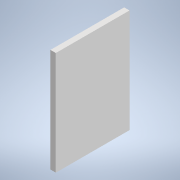
# Autodesk Inventor part: backPlate
Saved by Autodesk Inventor 2021.2 (Build 252289000, 289)
## iProperties
Created: 2021-02-12
Part Number: backPlate
Material: PC/ABS Plastic
Document SubType Name: Modeling
Designer: robst
Density: 0.357273 g/cm^3
Appearance: Smooth - White
Author: robst
Autodesk Inventor part; units mm, degrees
ref_plane "YZ Plane" through (0, 0, 0) normal (1, 0, 0) x (0, 1, 0)
ref_plane "XZ Plane" through (0, 0, 0) normal (0, 1, 0) x (-1, 0, 0)
ref_plane "XY Plane" through (0, 0, 0) normal (0, 0, 1) x (1, 0, 0)
sketch "Sketch1" plane through (0, 0, 0) normal (1, 0, 0) x (0, 1, 0)
  line L0 (-18.3138, 13.0328) -> (-18.3138, -13.0328)
  line L1 (-18.3138, -13.0328) -> (18.3138, -13.0328)
  line L2 (18.3138, -13.0328) -> (18.3138, 13.0328)
  line L3 (18.3138, 13.0328) -> (-18.3138, 13.0328)
  line L4 (-18.3138, 13.0328) -> (18.3138, -13.0328) construction
  line L5 (-18.3138, -13.0328) -> (18.3138, 13.0328) construction
  point P0 (0, 0)
  constraints: 12 end point, 2 midpoint, 2 parallel, 1 perpendicular, 1 vertical
extrude "Extrusion1" add sketch "Sketch1" against normal blind 1.905
body "Solid1"
